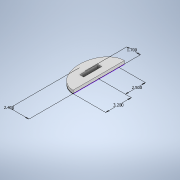
# Autodesk Inventor part: pryBarHolder
Saved by Autodesk Inventor 2021 (Build 250183000, 183)
## iProperties
Created: 2020-06-10
Part Number: pryBarHolder
Material: Generic
Document SubType Name: Modeling
Designer: robst
Density: 1 g/cm^3
Appearance: Default
Author: robst
Autodesk Inventor part; units mm, degrees
ref_plane "YZ Plane" through (0, 0, 0) normal (1, 0, 0) x (0, 1, 0)
ref_plane "XZ Plane" through (0, 0, 0) normal (0, 1, 0) x (-1, 0, 0)
ref_plane "XY Plane" through (0, 0, 0) normal (0, 0, 1) x (1, 0, 0)
sketch "Sketch1" plane through (0, 0, 0) normal (0, 1, 0) x (-1, 0, 0)
  ellipse E0 centre (0, 0) end of major axis (0, -81.28) minor radius 60.96 (0, -81.28) -> (0, 81.28) ccw
  line L0 (0, 81.28) -> (0, -81.28)
  ellipse E1 centre (0, 0) end of major axis (0, -63.5) minor radius 43.18 (0, -63.5) -> (0, 63.5) ccw
  line L1 (0, 81.28) -> (0, -81.28)
  dimension "d0" = 60.96
  dimension "d1" = 81.28
  dimension "d2" = 43.18
  dimension "d3" = 63.5
  constraints: 4 end point, 2 coincident, 2 point on line, 2 vertical, 8 other
extrude "Extrusion1" add sketch "Sketch1" along normal blind 9.525
extrude "Extrusion2" add sketch "Sketch1" against normal blind 9.525 contours L0 E1
sketch "Sketch3" plane through (0, -9.525, 0) normal (0, -1, 0) x (1, 0, 0)
  line L0 (0, -63.5) -> (0, 63.5) projected
  ellipse E0 centre (0, 0) end of major axis (0, -63.5) minor radius 43.18 (0, 63.5) -> (0, -63.5) ccw projected
  line L1 (0, 81.28) -> (0, -81.28) projected
  ellipse E1 centre (0, 0) end of major axis (0, -63.5) minor radius 43.18 (0, 63.5) -> (0, -63.5) ccw projected
  line L2 (-9.525, 61.9358) -> (-9.525, -61.9358)
  ellipse E2 centre (0, 0) end of major axis (0, -63.5) minor radius 43.18 (0, 63.5) -> (-9.525, 61.9358) ccw
  ellipse E3 centre (0, 0) end of major axis (0, -63.5) minor radius 43.18 (-9.525, -61.9358) -> (0, -63.5) ccw
  dimension "d8" = 9.525
  constraints: 4 vertical, 2 end point, 2 point on line, 1 coincident, 12 other
  measures "d8" distance between parallel lines of L2 L0
extrude "Extrusion3" cut sketch "Sketch3" against normal blind 9.525 contours E0 L2 L0
sketch "Sketch4" plane through (0, 9.525, 0) normal (0, 1, 0) x (1, 0, 0)
  line L0 (-19.05, -28.575) -> (-19.05, 28.575)
  line L1 (-19.05, 28.575) -> (-31.75, 28.575)
  line L2 (-31.75, 28.575) -> (-31.75, -28.575)
  line L3 (-31.75, -28.575) -> (-19.05, -28.575)
  line L4 (-19.05, -28.575) -> (-31.75, 28.575) construction
  line L5 (-19.05, 28.575) -> (-31.75, -28.575) construction
  ellipse E0 centre (0, 0) end of major axis (0, 63.5) minor radius 43.18 (-9.525, 61.9358) -> (-9.525, -61.9358) ccw projected
  line L6 (-19.05, 0) -> (-31.75, 0) construction
  ellipse E1 centre (0, 0) end of major axis (0, 81.28) minor radius 60.96 (0, 81.28) -> (0, -81.28) ccw construction
  line L7 (0, 0) -> (-60.96, 0) construction
  line L8 (0, -81.28) -> (0, 81.28) projected
  point P0 (-25.4, 0)
  dimension "d11" = 12.7
  dimension "d12" = 57.15
  dimension "d13" = 25.4
  constraints: 16 end point, 4 midpoint, 2 parallel, 1 collinear, 1 horizontal, 1 perpendicular, 1 vertical, 4 other
  measures "d11" distance of L2.end L0.start
  measures "d12" distance of L1.end L2.end
  measures "d13" distance from line of point (-25.4, 0) L8
extrude "Extrusion4" cut sketch "Sketch4" against normal through all
body "Solid1"
